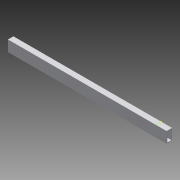
# Autodesk Inventor part: Arm
Saved by Autodesk Inventor 2015 (Build 190159000, 159)
## iProperties
Created: 2015-01-11
Part Number: Arm
Material: Aluminum 6061
Document SubType Name: Modeling
Designer: chapale16
Density: 2.7 g/cm^3
Appearance: Aluminum - Flat
Author: chapale16
Autodesk Inventor part; units mm, degrees
ref_plane "YZ Plane" through (0, 0, 0) normal (1, 0, 0) x (0, 1, 0)
ref_plane "XZ Plane" through (0, 0, 0) normal (0, 1, 0) x (-1, 0, 0)
ref_plane "XY Plane" through (0, 0, 0) normal (0, 0, 1) x (1, 0, 0)
sketch "Sketch1" plane through (0, 0, 0) normal (0, 1, 0) x (-1, 0, 0)
  line L0 (0, 25.4) -> (685.8, 25.4)
  line L1 (0, 0) -> (685.8, 0)
  line L2 (685.8, 0) -> (685.8, 25.4)
  line L3 (0, 0) -> (-50.8, 0)
  line L4 (0, 25.4) -> (-50.8, 25.4)
  line L5 (-50.8, 25.4) -> (-50.8, 0)
  dimension "d0" = 25.4
  dimension "d1" = 685.8
  dimension "d20" = 50.8
  constraints: 12 end point, 2 horizontal
  measures "d0" distance of L1.start L0.start
  measures "d1" distance of L0.start L0.end
  measures "d20" distance of L0.start L4.end
extrude "Extrusion1" add sketch "Sketch1" along normal blind 50.8
sketch "Sketch6" plane through (50.8, 0, 25.4) normal (1, 0, 0) x (0, 0, -1)
  line L0 (0, 50.8) -> (0, 0)
  line L1 (0, 0) -> (25.4, 0)
  line L2 (25.4, 0) -> (25.4, 50.8)
  line L3 (25.4, 50.8) -> (0, 50.8)
  line L4 (25.4, 50.8) -> (0, 50.8) projected
  line L5 (3.1242, 47.6758) -> (3.1242, 3.1242)
  line L6 (3.1242, 3.1242) -> (22.2758, 3.1242)
  line L7 (22.2758, 3.1242) -> (22.2758, 47.6758)
  line L8 (22.2758, 47.6758) -> (3.1242, 47.6758)
  dimension "d21" = 3.1242
  constraints: 16 end point, 4 perpendicular, 1 collinear, 1 vertical, 3 other
  measures "d21" distance between parallel lines of L3 L8
extrude "Extrusion4" cut sketch "Sketch6" against normal blind 736.6 contours L8 L7 L6 L5
sketch "Sketch7" plane through (0, 50.8, 0) normal (0, 1, 0) x (1, 0, 0)
  point P0 (0, 0)
  point P1 (0, -12.7)
body "Solid1"
